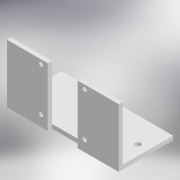
# Autodesk Inventor part: horizontal_axis_motor_metal_holder
Saved by Autodesk Inventor 2021 (Build 250183000, 183)
## iProperties
Created: 2020-10-10
Part Number: horizontal_axis_motor_metal_holder
Material: Generic
Document SubType Name: Modeling
Designer: bober
Density: 1 g/cm^3
Appearance: Default
Author: bober
Autodesk Inventor part; units mm, degrees
ref_plane "YZ Plane" through (0, 0, 0) normal (1, 0, 0) x (0, 1, 0)
ref_plane "XZ Plane" through (0, 0, 0) normal (0, 1, 0) x (-1, 0, 0)
ref_plane "XY Plane" through (0, 0, 0) normal (0, 0, 1) x (1, 0, 0)
sketch "Sketch1" plane through (0, 0, 0) normal (0, 1, 0) x (-1, 0, 0)
  line L0 (-21, 18.5) -> (21, 18.5)
  line L1 (21, 18.5) -> (21, -18.5)
  line L2 (21, -18.5) -> (-21, -18.5)
  line L3 (-21, -18.5) -> (-21, 18.5)
  line L4 (-21, 18.5) -> (21, -18.5) construction
  line L5 (21, 18.5) -> (-21, -18.5) construction
  point P0 (0, 0)
  dimension "d0" = 42
  dimension "d1" = 37
  constraints: 12 end point, 2 midpoint, 2 parallel, 1 horizontal, 1 perpendicular
  measures "d0" distance of L1.end L2.end
  measures "d1" distance of L0.end L1.end
extrude "Extrusion1" add sketch "Sketch1" along normal blind 3
sketch "Sketch2" plane through (-21, 0, 18.5) normal (0, 0, 1) x (1, 0, 0)
  line L0 (42, 0) -> (0, 0) projected
  line L1 (0, 0) -> (10, 0)
  line L2 (10, 0) -> (10, 45)
  line L3 (10, 45) -> (0, 45)
  line L4 (0, 45) -> (0, 0)
  point P0 (21, 0)
  dimension "d4" = 10
  dimension "d5" = 45
  constraints: 8 end point, 2 parallel, 1 horizontal, 1 perpendicular
  measures "d4" distance of L3.end L2.end
  measures "d5" distance of L2.end L1.end
extrude "Extrusion2" add sketch "Sketch2" along normal blind 3
sketch "Sketch3" plane through (-21, 0, 21.5) normal (0, 0, 1) x (1, 0, 0)
  circle A0 centre (5, 40) radius 1.5
  circle A1 centre (5, 8) radius 1.5
  point P0 (21, 0)
  dimension "d8" = 3
  dimension "d9" = 3
  constraints: 2 centre point
  measures "d8" diameter of A0
  measures "d9" diameter of A1
extrude "Extrusion3" cut sketch "Sketch3" against normal blind 3
thicken "Thicken2" operation add thickness 20 both sides no extend neighbours yes toward (-1, 0, 0) faces at (-21, 16, 20.5)
mirror "Mirror3" about plane through (0, 0, 0) normal (1, 0, 0) of "Extrusion2", "Extrusion3"
thicken "Thicken3" operation add thickness 20 both sides no extend neighbours yes toward (1, 0, 0) faces at (21, 16, 20.5)
sketch "Sketch8" plane through (0, 3, 0) normal (0, 1, 0) x (1, 0, 0)
  circle A0 centre (33.5, 0) radius 2
  circle A1 centre (-33.5, 0) radius 2
  point P0 (0, 0)
  dimension "d28" = 4
  dimension "d29" = 4
  constraints: 2 centre point
  measures "d28" diameter of A0
  measures "d29" diameter of A1
extrude "Extrusion6" cut sketch "Sketch8" against normal blind 10
thicken "Thicken4" operation add thickness 2 both sides no extend neighbours yes toward (0, -1, 0) faces at (-21, 45, 20.5)
thicken "Thicken5" operation add thickness 2 both sides no extend neighbours yes toward (0, -1, 0) faces at (21, 45, 20.5)
body "Solid1"
